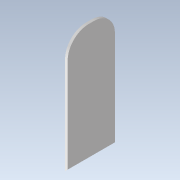
# Autodesk Inventor part: platina_3
Saved by Autodesk Inventor 2021 (Build 250183000, 183)
## iProperties
Created: 2021-04-25
Part Number: platina_3
Material: Genérico
Document SubType Name: Modeling
Designer: j2seb
Density: 1 g/cm^3
Appearance: Valor por defecto
Author: j2seb
Autodesk Inventor part; units mm, degrees
ref_plane "YZ Plane" through (0, 0, 0) normal (1, 0, 0) x (0, 1, 0)
ref_plane "XZ Plane" through (0, 0, 0) normal (0, 1, 0) x (-1, 0, 0)
ref_plane "XY Plane" through (0, 0, 0) normal (0, 0, 1) x (1, 0, 0)
sketch "Boceto1" plane through (0, 0, 0) normal (1, 0, 0) x (0, 1, 0)
  line L0 (0, 0) -> (45, 0)
  line L1 (45, 0) -> (45, -18)
  line L2 (45, -18) -> (0, -18)
  line L3 (0, -18) -> (0, 0)
  dimension "d2" = 45
  dimension "d3" = 18
  constraints: 8 end point, 2 parallel, 1 horizontal, 1 perpendicular
  measures "d2" distance of L1.end L2.end
  measures "d3" distance between parallel lines of L2 L0
extrude "Extrusión1" add sketch "Boceto1" along normal blind 1
chamfer "Chaflán1" distance 1 angle 45 1 edges at (1, 0, -9)
fillet "Empalme1" radius 8 2 edges at (0.5, 45, -18) (0.5, 45, 0)
sketch "Boceto2" plane through (1, 0, 0) normal (1, 0, 0) x (0, 0, -1)
  point P0 (6.124, 36.1455)
hole "Agujero1" at (1, 36.1455, -6.124) direction (-1, 0, 0) diameter 3.4 end through all
